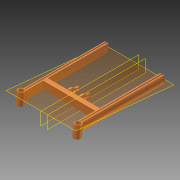
# Autodesk Inventor part: frame
Saved by Autodesk Inventor 2012 (Build 160160000, 160)
## iProperties
Created: 2012-03-07
Part Number: frame
Material: Default
Document SubType Name: Modeling
Designer: esv
Density: 1 g/cm^3
Author: esv
Autodesk Inventor part; units mm, degrees
note: some values were not read from the file. Chosen so that the rebuilt part matches the saved one: sketch regions of "Bracket".
ref_plane "YZ Plane" through (0, 0, 0) normal (1, 0, 0) x (0, 1, 0)
ref_plane "XZ Plane" through (0, 0, 0) normal (0, 1, 0) x (-1, 0, 0)
ref_plane "XY Plane" through (0, 0, 0) normal (0, 0, 1) x (1, 0, 0)
sketch "Sketch1" plane through (0, 0, 0) normal (0, 0, 1) x (1, 0, 0)
  line L0 (0, 0) -> (0, 60.325)
  line L1 (0, 60.325) -> (23.7924, 60.325)
  line L2 (23.7924, 0) -> (0, 0)
  arc A0 (26.383, 1.3393) -> (26.383, 58.9857) centre (-14.2925, 30.1625) ccw
  arc A1 (26.383, 58.9857) -> (23.7924, 60.325) centre (23.7924, 57.15) ccw
  arc A2 (23.7924, 0) -> (26.383, 1.3393) centre (23.7924, 3.175) ccw
  line L3 (35.56, 22.9711) -> (35.56, 50.1168)
  line L4 (8.636, 60.325) -> (18.3388, 60.325)
  line L5 (18.3388, 60.325) -> (18.3388, 47.2694)
  line L6 (18.3388, 47.2694) -> (8.636, 47.2694)
  line L7 (8.636, 47.2694) -> (8.636, 60.325)
  line L8 (21.9964, 56.515) -> (4.9784, 56.515)
  line L9 (4.9784, 56.515) -> (4.9784, 47.2694)
  line L10 (4.9784, 47.2694) -> (21.9964, 47.2694)
  line L11 (21.9964, 47.2694) -> (21.9964, 56.515)
  point P0 (25.4, 60.325)
  point P1 (25.4, 0)
  point P2 (13.4874, 47.2694)
  dimension "d1" = 60.325
  dimension "d3" = 25.4
  dimension "d4" = 3.175
  dimension "d5" = 35.56
  dimension "d6" = 8.636
  dimension "d7" = 9.7028
  dimension "d8" = 13.0556
  dimension "d9" = 3.81
  dimension "d10" = 17.018
  constraints: 24 end point, 8 point on circle, 6 parallel, 5 tangent, 4 perpendicular, 3 centre point, 3 point on line, 2 horizontal, 2 midpoint, 1 equal radius, 1 vertical
  measures "d1" distance of L0.start L0.end
  measures "d3" distance of point (25.4, 0) L0.start
  measures "d4" radius of A1
  measures "d5" distance between parallel lines of L0 L3
  measures "d6" distance between parallel lines of L0 L7
  measures "d7" distance between parallel lines of L7 L5
  measures "d8" distance between parallel lines of L6 L1
  measures "d9" distance between parallel lines of L8 L1
  measures "d10" distance of L9.end L10.end
extrude "Side Rail" add sketch "Sketch1" along normal blind 622.3 contours L0 L1 L7 L8 L9 L10 L6 L11 L5 A1 A0 A2 L2
sketch "Sketch5" plane through (0, 0, 0) normal (-1, 0, 0) x (0, 0, 1)
  line L0 (0, 60.325) -> (622.3, 60.325) projected
  line L1 (0, 60.325) -> (0, 0) projected
  line L2 (0, 0) -> (622.3, 0) projected
  line L3 (460.375, 60.325) -> (488.95, 60.325)
  line L4 (492.125, 57.15) -> (492.125, 3.175)
  line L5 (488.95, 0) -> (460.375, 0)
  line L6 (457.2, 3.175) -> (457.2, 57.15)
  arc A0 (460.375, 60.325) -> (457.2, 57.15) centre (460.375, 57.15) ccw
  arc A1 (457.2, 3.175) -> (460.375, 0) centre (460.375, 3.175) ccw
  arc A2 (492.125, 57.15) -> (488.95, 60.325) centre (488.95, 57.15) ccw
  arc A3 (488.95, 0) -> (492.125, 3.175) centre (488.95, 3.175) ccw
  point P0 (457.2, 60.325)
  point P1 (492.125, 0)
  dimension "d24" = 34.925
  dimension "d25" = 3.175
  dimension "d26" = 457.2
  constraints: 8 end point, 8 point on circle, 8 tangent, 6 point on line, 4 centre point, 3 equal radius, 2 parallel, 1 horizontal, 1 perpendicular
  measures "d24" distance between parallel lines of L6 L4
  measures "d25" radius of A0
  measures "d26" distance between parallel lines of L6 L1
extrude "Cross Bar" add sketch "Sketch5" along normal blind 393.7 contours L0 A2 L4 A3 L2 A1 L6 A0
ref_plane "Work Plane1" through (-196.85, 60.325, 488.95) normal (1, 0, 0) x (0, 1, 0)
ref_plane "Work Plane2" through (-147.8026, 60.325, 488.95) normal (1, 0, 0) x (0, 1, 0)
sketch "Sketch6" plane through (-147.8026, 60.325, 488.95) normal (1, 0, 0) x (0, 1, 0)
  line L0 (1.9304, -31.75) -> (-62.2554, -31.75)
  line L1 (-62.2554, -31.75) -> (-62.2554, -57.15)
  line L2 (1.9304, -56.2046) -> (1.9304, -31.75)
  line L3 (-57.15, -31.75) -> (-3.175, -31.75)
  line L4 (1.4132, -57.9414) -> (-13.6341, -80.9671)
  line L5 (-14.6685, -84.4409) -> (-14.6685, -107.95)
  line L6 (-14.6685, -107.95) -> (-26.8605, -107.95)
  line L7 (-26.8605, -107.95) -> (-26.8605, -85.5076)
  line L8 (-30.1625, -31.75) -> (-30.1625, -153.8452)
  arc A0 (-26.8605, -77.9122) -> (-33.4645, -77.9122) centre (-30.1625, -69.85) ccw
  arc A1 (1.4132, -57.9414) -> (1.9304, -56.2046) centre (-1.2446, -56.2046) ccw
  line L9 (-11.43, -31.75) -> (-48.895, -31.75)
  line L10 (-48.895, -31.75) -> (-48.895, -51.2412)
  line L11 (-11.43, -51.2412) -> (-11.43, -31.75)
  arc A2 (-21.2978, -56.5278) -> (-11.43, -51.2412) centre (-17.78, -51.2412) ccw
  arc A3 (-13.6341, -80.9671) -> (-14.6685, -84.4409) centre (-8.3185, -84.4409) ccw
  line L12 (-61.7382, -57.9414) -> (-46.6909, -80.9671)
  line L13 (-45.6565, -84.4409) -> (-45.6565, -107.95)
  line L14 (-45.6565, -107.95) -> (-33.4645, -107.95)
  line L15 (-33.4645, -107.95) -> (-33.4645, -77.9122)
  arc A4 (-62.2554, -56.2046) -> (-61.7382, -57.9414) centre (-59.0804, -56.2046) ccw
  arc A5 (-45.6565, -84.4409) -> (-46.6909, -80.9671) centre (-52.0065, -84.4409) ccw
  arc A6 (-48.895, -51.2412) -> (-39.0272, -56.5278) centre (-42.545, -51.2412) ccw
  line L16 (-45.6565, -57.15) -> (-44.8708, -57.15)
  line L17 (-40.2192, -57.15) -> (-39.8977, -57.15)
  line L18 (-62.2554, -57.15) -> (-62.1114, -57.15)
  line L19 (-40.2192, -57.15) -> (-39.8977, -57.15)
  line L20 (1.7864, -57.15) -> (1.9304, -57.15)
  arc A7 (-21.2978, -56.5278) -> (-39.8977, -57.15) centre (-30.1625, -69.85) ccw
  line L21 (-26.8605, -85.5076) -> (-26.8605, -77.9122)
  line L22 (-14.6685, -107.95) -> (-14.6685, -84.4409)
  line L23 (-16.8821, -107.95) -> (-14.6685, -84.4409)
  point P0 (-60.325, -488.95)
  point P1 (-14.6685, -82.55)
  point P2 (-33.4645, -77.9122)
  dimension "d30" = 64.1858
  dimension "d31" = 25.4
  dimension "d32" = 3.175
  dimension "d33" = 17.4244
  dimension "d34" = 13.3604
  dimension "d35" = 38.1
  dimension "d36" = 12.192
  dimension "d37" = 15.494
  dimension "d39" = 6.35
  dimension "d40" = 76.2
  dimension "d41" = 25.4
  dimension "d42" = 6.35
  dimension "d43" = 6.35
  dimension "d44" = 16.002
  dimension "d45" = 25.4
  dimension "d46" = 25.4
  dimension "d47" = 25.4
  dimension "d48" = 46.1622
  dimension "d49" = 122.0952
  dimension "d50" = 30.0378
  dimension "d61" = 5.379
  constraints: 48 end point, 21 point on circle, 9 point on line, 9 symmetric about line, 9 tangent, 8 centre point, 8 parallel, 5 perpendicular, 3 midpoint, 2 horizontal, 1 coincident, 2 other
  measures "d30" distance of L0.start L0.end
  measures "d31" distance of L20.end L0.start
  measures "d32" radius of A1
  measures "d33" diameter of A0
  measures "d34" distance between parallel lines of L2 L11
  measures "d35" distance from line of L0 A7.centre
  measures "d36" distance of L5.end L6.end
  measures "d37" distance between parallel lines of L8 L5
  measures "d39" radius of A2
  measures "d40" distance between parallel lines of L0 L6
  measures "d41" distance of point (-14.668, -82.55) L5.end
  measures "d42" radius of A3
  measures "d43" radius of A6
  measures "d44" radius of A7
  measures "d45" distance between parallel lines of L19 L3
  measures "d46" distance between parallel lines of L16 L3
  measures "d47" distance between parallel lines of L18 L3
  measures "d48" distance from line of L21.end L3
  measures "d49" distance from line of L8.end L3
  measures "d50" distance of L14.end L15.end
  measures "d61" angle of L23 L5
extrude "Bracket" add sketch "Sketch6" against normal blind 12.7 contours L2 A1 L4 A3 L23 L6 L7 L21 A0 L8 A7 A2 L11 L0 | L10 A6 L17 A7 L8 A0 L15 L14 L13 A5 L12 A4 L1 L0 | L5 L6 L23 | A4 L18 L1
sketch "Sketch7" plane through (-147.8026, 45.6565, 404.5091) normal (0, 1, 0) x (1, 0, 0)
  line L0 (0, 23.5091) -> (-12.7, 23.5091) projected
  point P0 (147.8026, 404.5091)
  point P1 (-6.35, 16.6511)
  point P2 (-6.35, 23.5091)
  dimension "d53" = 6.858
  constraints: 1 midpoint, 1 vertical alignment
  measures "d53" distance from line of L0 point (-6.35, 16.651)
hole "Hole1" at (-154.1526, 45.6565, 387.858) direction (0, -1, 0) diameter 6.35 end through all
sketch "Sketch8" plane through (0, 0, 0) normal (-1, 0, 0) x (0, 0, 1)
  line L0 (0, 60.325) -> (0, 0) projected
  point P0 (28.575, 30.1625)
  point P1 (0, 30.1625)
  dimension "d62" = 28.575
  constraints: 1 horizontal alignment, 1 midpoint
  measures "d62" distance from line of L0 point (28.575, 30.162)
hole "Hole2" at (0, 30.1625, 28.575) direction (1, 0, 0) diameter 6.35 end through all
ref_plane "Work Plane5" through (-417.4924, 60.325, 622.3) normal (0, 0.9955964, -0.0937434) x (-1, 0, 0)
sketch "Sketch9" plane through (-417.4924, 60.325, 622.3) normal (0, 0.9955964, -0.0937434) x (-1, 0, 0)
  circle A0 centre (-435.8312, 19.05) radius 25.4
  circle A1 centre (-435.8312, 19.05) radius 18.034
  line L0 (-435.8312, -619.5596) -> (-435.8312, 0) projected
  line L1 (-417.4924, 0) -> (-441.2849, 0) projected
  point P0 (-417.4924, -625.2147)
  point P1 (-435.8312, -6.3155)
  point P2 (-418.4519, 0)
  dimension "d71" = 50.8
  dimension "d72" = 7.366
  dimension "d73" = 19.05
  constraints: 2 centre point, 1 coincident, 1 point on line
  measures "d71" diameter of A0
  measures "d72" radial gap between concentric circles of A0 A1
  measures "d73" distance from line of A0.centre L1
extrude "Extrusion5" add sketch "Sketch9" against normal blind 88.9
mirror "Mirror5" about plane through (-196.85, 60.325, 488.95) normal (1, 0, 0) of "Extrusion5", "Side Rail", "Bracket", "Hole2"
body "Solid1"
